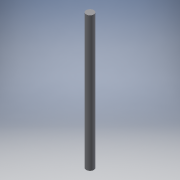
# Autodesk Inventor part: GuiaLinear_12x200mm
Saved by Autodesk Inventor 2018 (Build 220112000, 112)
## iProperties
Created: 2018-07-23
Part Number: GuiaLinear_12x200mm
Material: Genérico
Document SubType Name: Modeling
Designer: Usuario
Density: 1 g/cm^3
Appearance: Padrão
Mass: 22.6195 g
Surface Area: 77.6602 cm^2
Volume: 22.6195 cm^3
Author: Usuario
Autodesk Inventor part; units mm, degrees
ref_plane "YZ Plane" through (0, 0, 0) normal (1, 0, 0) x (0, 1, 0)
ref_plane "XZ Plane" through (0, 0, 0) normal (0, 1, 0) x (-1, 0, 0)
ref_plane "XY Plane" through (0, 0, 0) normal (0, 0, 1) x (1, 0, 0)
sketch "Esboço1" plane through (0, 0, 0) normal (0, 0, 1) x (1, 0, 0)
  circle A0 centre (0, 0) radius 6
  dimension "d0" = 12
  constraints: 1 centre point, 1 coincident
  measures "d0" diameter of A0
extrude "Extrusão1" add sketch "Esboço1" along normal blind 210
